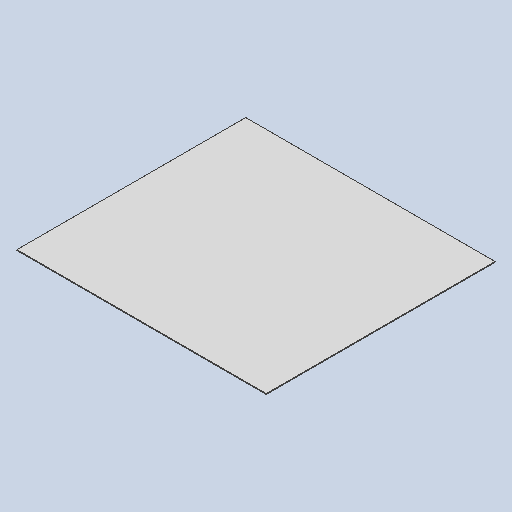
# Autodesk Inventor part: GBK bottom 0124
Saved by Autodesk Inventor 2026.2 (Build 302298000, 298)
## iProperties
Created: 2026-05-19
Part Number: GBK bottom 0124
Material: Steel
Document SubType Name: Sheet Metal
Designer: user
Density: 7.85 g/cm^3
Sheet Metal Rule: Default_mm
Appearance: Default
Mass: 88312.5 g
Surface Area: 45300 cm^2
Volume: 11250 cm^3
Flat Pattern Width: 148 cm
Flat Pattern Length: 161.3 cm
Flat Pattern Area: 23872.4 cm^2
Sheet Metal Width: 1480,000 mm
Sheet Metal Length: 1613,000 mm
Sheet Metal Area: 2387240,000 mm^2
Author: user
Autodesk Inventor part; units mm, degrees
ref_plane "YZ Plane" through (0, 0, 0) normal (1, 0, 0) x (0, 1, 0)
ref_plane "XZ Plane" through (0, 0, 0) normal (0, 1, 0) x (-1, 0, 0)
ref_plane "XY Plane" through (0, 0, 0) normal (0, 0, 1) x (1, 0, 0)
sketch "Эскиз1" plane through (0, 0, 0) normal (0, 1, 0) x (-1, 0, 0)
  line L0 (806.5, 740) -> (-806.5, 740)
  line L1 (-806.5, 740) -> (-806.5, -740)
  line L2 (-806.5, -740) -> (806.5, -740)
  line L3 (806.5, -740) -> (806.5, 740)
  line L4 (806.5, 740) -> (-806.5, -740) construction
  line L5 (-806.5, 740) -> (806.5, -740) construction
  point P0 (0, 0)
  dimension "d0" = 1613
  dimension "d1" = 1480
  measures "d0" distance of L2.end L1.end
  measures "d1" distance of L1.end L0.end
extrude "Пластина1" add sketch "Эскиз1" along normal blind 5
equation "\"d2\" = Толщина"
equation "\"Радиус_гибки\" = Толщина"
equation "\"Ширина_просечки\" = Толщина"
equation "\"Глубина_просечки\" = 0.5 * Толщина"
equation "\"Радиус_перехода\" = Радиус_гибки"
equation "\"Радиус_Якоби\" = Радиус_гибки"
equation "\"Размер_зазора\" = Толщина"
equation "\"Толщина\" = 5"
